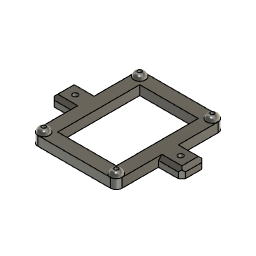
ELE#DLC_holder (Autodesk Fusion 360 design; units mm, degrees)
Autodesk Fusion 360 part; units mm, degrees
sketch "Sketch1" plane through (0, 0, 0) normal (0, 0, 1) x (1, 0, 0)
  line L0 (0, 0) -> (70, 0)
  line L1 (70, 0) -> (70, 90)
  line L2 (70, 90) -> (0, 90)
  line L3 (0, 90) -> (0, 0)
  line L4 (66.000001, 90) -> (4.000001, 90)
  line L5 (0, 90) -> (0, 86.000001)
  line L6 (0, 86.000001) -> (0, 4.000001)
  line L7 (0, 86.000001) -> (70, 86.000001)
  line L8 (66.000001, 90) -> (66.000001, 86.000001)
  line L9 (66.000001, 84.000001) -> (66.000001, 0)
  line L10 (4, 86.000001) -> (4, 0)
  line L11 (0, 4.000001) -> (4, 4.000001)
  line L12 (66.000001, 4) -> (70, 4)
  circle A0 centre (4, 86.000001) radius 1.75
  circle A1 centre (66.000001, 86.000001) radius 1.75
  circle A2 centre (66.000001, 4) radius 1.75
  circle A3 centre (4, 4.000001) radius 1.75
  dimension "d1" = 70
  dimension "d2" = 90
  dimension "d5" = 3.5
  dimension "d6" = 3.5
  dimension "d7" = 3.5
  dimension "d8" = 3.5
  constraint horizontal L0
  constraint vertical L1
  constraint horizontal L2
  constraint vertical L3
  constraint coincident L0.start L3.end
  constraint perpendicular L1 L4
  constraint perpendicular L2 L6
  constraint perpendicular L1 L7
  constraint perpendicular L7 L8
  constraint perpendicular L0 L9
  constraint coincident L0 L10.end
  constraint perpendicular L0 L10
  constraint perpendicular L10 L11
  constraint coincident L1 L12.end
  constraint perpendicular L1 L12
  measures "d1" distance of L0.start L0.end
  measures "d2" distance of L0.start L2.end
  measures "d5" diameter of A0
  measures "d6" diameter of A1
  measures "d7" diameter of A2
  measures "d8" diameter of A3
extrude "Extrude1" add sketch "Sketch1" along normal blind 8 contours L0 L3 L10 L11 A3 | L0 L1 L7 L9 L10 L12 A0 A1 A2 A3 | L3 L6 L7 L10 L11 A0 A3 | L0 L1 L9 L12 A2 | L2 L3 L4 L5 L7 L8 A0 A1 | L1 L2 L7 L8 A1 picked at (2.351293, 0.842603) picked at (25.066969, 58.2106) picked at (1.091008, 58.136049) picked at (67.648708, 0.842602) picked at (25.192233, 88.919766) picked at (69.157398, 87.648708)
sketch "Sketch2" plane through (0, 0, 0) normal (0, 0, -1) x (1, 0, 0)
  circle A0 centre (66.000001, -86.000001) radius 1.75
  circle A1 centre (4, -4.000001) radius 1.75
  circle A2 centre (4, -86.000001) radius 1.75
  circle A3 centre (66.000001, -4) radius 1.75
  line L0 (0, 0) -> (0, -90)
  line L1 (0, -90) -> (70, -90)
  line L2 (70, -90) -> (70, 0)
  line L3 (70, 0) -> (0, 0)
  line L4 (6.8, -2.383421) -> (4, -0.76684)
  line L5 (4, -0.76684) -> (1.2, -2.383421)
  line L6 (1.2, -2.383421) -> (1.2, -5.616582)
  line L7 (1.2, -5.616582) -> (4, -7.233163)
  line L8 (4, -7.233163) -> (6.8, -5.616582)
  line L9 (6.8, -5.616582) -> (6.8, -2.383421)
  line L10 (63.200001, -5.616581) -> (66.000001, -7.233162)
  line L11 (66.000001, -7.233162) -> (68.800001, -5.616581)
  line L12 (68.800001, -5.616581) -> (68.800001, -2.383419)
  line L13 (68.800001, -2.383419) -> (66.000001, -0.766839)
  line L14 (66.000001, -0.766839) -> (63.200001, -2.383419)
  line L15 (63.200001, -2.383419) -> (63.200001, -5.616581)
  line L16 (63.200001, -87.616582) -> (66.000001, -89.233163)
  line L17 (66.000001, -89.233163) -> (68.800001, -87.616582)
  line L18 (68.800001, -87.616582) -> (68.800001, -84.383421)
  line L19 (68.800001, -84.383421) -> (66.000001, -82.76684)
  line L20 (66.000001, -82.76684) -> (63.200001, -84.383421)
  line L21 (63.200001, -84.383421) -> (63.200001, -87.616582)
  line L22 (6.8, -84.383421) -> (4, -82.76684)
  line L23 (4, -82.76684) -> (1.2, -84.383421)
  line L24 (1.2, -84.383421) -> (1.2, -87.616582)
  line L25 (1.2, -87.616582) -> (4, -89.233163)
  line L26 (4, -89.233163) -> (6.8, -87.616582)
  line L27 (6.8, -87.616582) -> (6.8, -84.383421)
  point P0 (4, -4.000001)
  point P1 (66.000001, -4)
  point P2 (66.000001, -86.000001)
  point P3 (4, -86.000001)
  dimension "d11" = 2.8
  dimension "d12" = 2.8
  dimension "d13" = 2.8
  dimension "d14" = 2.8
extrude "Extrude2" cut sketch "Sketch2" against normal blind 8 contours A2 | L4 L5 L6 L7 L8 L9 | L10 L11 L12 L13 L14 L15 | L16 L17 L18 L19 L20 L21 | L22 L23 L24 L25 L26 L27 picked at (4.363702, -86.962267) picked at (5.225, -1.878239) picked at (64.775001, -1.878238) picked at (64.775001, -88.121764) picked at (2.775, -83.878239)
extrude "Extrude3" add 1 faces at (46.666667, 90, 5.333333) along direction (0, 1, 0) blind 1
extrude "Extrude4" add 1 faces at (70, 30.333333, 2.666667) along direction (1, 0, 0) blind 1
extrude "Extrude5" add 1 faces at (0, 30.333333, 2.666667) along direction (-1, 0, 0) blind 1
extrude "Extrude6" add 1 faces at (23, 0, 5.333333) along direction (0, -1, 0) blind 1
sketch "Sketch3" plane through (0, 0, 0) normal (0, 0, -1) x (1, 0, 0)
  line L0 (4, -0.76684) -> (6.8, -2.383421)
  line L1 (6.8, -2.383421) -> (6.8, -5.616582)
  line L2 (6.8, -5.616582) -> (4, -7.233163)
  line L3 (4, -7.233163) -> (1.2, -5.616582)
  line L4 (1.2, -5.616582) -> (1.2, -2.383421)
  line L5 (1.2, -2.383421) -> (4, -0.76684)
  line L6 (4, -82.76684) -> (6.8, -84.383421)
  line L7 (6.8, -84.383421) -> (6.8, -87.616582)
  line L8 (6.8, -87.616582) -> (4, -89.233163)
  line L9 (4, -89.233163) -> (1.2, -87.616582)
  line L10 (1.2, -87.616582) -> (1.2, -84.383421)
  line L11 (1.2, -84.383421) -> (4, -82.76684)
  line L12 (66.000001, -7.233162) -> (63.200001, -5.616581)
  line L13 (63.200001, -5.616581) -> (63.200001, -2.383419)
  line L14 (63.200001, -2.383419) -> (66.000001, -0.766839)
  line L15 (66.000001, -0.766839) -> (68.800001, -2.383419)
  line L16 (68.800001, -2.383419) -> (68.800001, -5.616581)
  line L17 (68.800001, -5.616581) -> (66.000001, -7.233162)
  line L18 (66.000001, -89.233163) -> (63.200001, -87.616582)
  line L19 (63.200001, -87.616582) -> (63.200001, -84.383421)
  line L20 (63.200001, -84.383421) -> (66.000001, -82.76684)
  line L21 (66.000001, -82.76684) -> (68.800001, -84.383421)
  line L22 (68.800001, -84.383421) -> (68.800001, -87.616582)
  line L23 (68.800001, -87.616582) -> (66.000001, -89.233163)
  line L24 (-1, -91) -> (71, -91)
  line L25 (71, -91) -> (71, 1)
  line L26 (71, 1) -> (-1, 1)
  line L27 (-1, 1) -> (-1, -91)
  line L28 (-1, -91) -> (71, 1)
  line L29 (35, -45) -> (35, -15)
  line L30 (35, -15) -> (60.000001, -15)
  line L31 (60.000001, -15) -> (60.000001, -75)
  line L32 (60.000001, -75) -> (10, -75)
  line L33 (10, -75) -> (10, -15)
  line L34 (10, -15) -> (35, -15)
  dimension "d25" = 60
  dimension "d26" = 60
  constraint coincident L24.start L27.end
  constraint coincident L25.end L26.start
  constraint midpoint L28 L29.start
  constraint parallel L16 L29
  constraint perpendicular L16 L30
  constraint perpendicular L30 L31
  constraint perpendicular L31 L32
  constraint perpendicular L32 L33
  constraint perpendicular L29 L34
  measures "d26" distance of L32.end L33.end
extrude "Extrude7" cut sketch "Sketch3" against normal blind 8 contours L28 L29 L32 L33 L34 | L28 L30 L31 L32 | L28 L29 L30 picked at (18.333333, -45) picked at (35.507247, -65) picked at (42.826087, -25)
sketch "Sketch4" plane through (0, 0, 8) normal (0, 0, 1) x (-1, 0, 0)
  line L0 (-10, -75) -> (-60.000001, -75)
  line L1 (-60.000001, -75) -> (-60.000001, -15)
  line L2 (-60.000001, -15) -> (-10, -15)
  line L3 (-10, -15) -> (-10, -75)
  line L4 (-6.8, -2.383421) -> (-4, -0.76684)
  line L5 (-4, -0.76684) -> (-1.2, -2.383421)
  line L6 (-1.2, -2.383421) -> (-1.2, -5.616582)
  line L7 (-1.2, -5.616582) -> (-4, -7.233163)
  line L8 (-4, -7.233163) -> (-6.8, -5.616582)
  line L9 (-6.8, -5.616582) -> (-6.8, -2.383421)
  line L10 (-6.8, -84.383421) -> (-4, -82.76684)
  line L11 (-4, -82.76684) -> (-1.2, -84.383421)
  line L12 (-1.2, -84.383421) -> (-1.2, -87.616582)
  line L13 (-1.2, -87.616582) -> (-4, -89.233163)
  line L14 (-4, -89.233163) -> (-6.8, -87.616582)
  line L15 (-6.8, -87.616582) -> (-6.8, -84.383421)
  line L16 (-63.200001, -5.616581) -> (-66.000001, -7.233162)
  line L17 (-66.000001, -7.233162) -> (-68.800001, -5.616581)
  line L18 (-68.800001, -5.616581) -> (-68.800001, -2.383419)
  line L19 (-68.800001, -2.383419) -> (-66.000001, -0.766839)
  line L20 (-66.000001, -0.766839) -> (-63.200001, -2.383419)
  line L21 (-63.200001, -2.383419) -> (-63.200001, -5.616581)
  line L22 (-63.200001, -87.616582) -> (-66.000001, -89.233163)
  line L23 (-66.000001, -89.233163) -> (-68.800001, -87.616582)
  line L24 (-68.800001, -87.616582) -> (-68.800001, -84.383421)
  line L25 (-68.800001, -84.383421) -> (-66.000001, -82.76684)
  line L26 (-66.000001, -82.76684) -> (-63.200001, -84.383421)
  line L27 (-63.200001, -84.383421) -> (-63.200001, -87.616582)
  line L28 (-71, 1) -> (-71, -91)
  line L29 (-71, -91) -> (1, -91)
  line L30 (1, -91) -> (1, 1)
  line L31 (1, 1) -> (-71, 1)
  circle A0 centre (-4, -86.000001) radius 5
  circle A1 centre (-66.000001, -86.000001) radius 4.999999
  circle A2 centre (-66.000001, -4) radius 5
  circle A3 centre (-4, -4) radius 5
  constraint tangent L30 A0
  constraint tangent L28 A1
  constraint tangent L30 A3
extrude "Extrude8" add sketch "Sketch4" along normal blind 4 contours A2 | A1 | A3 | A0 picked at (-64.233334, -7.059957) picked at (-69.533334, -86.000001) picked at (-0.466667, -4.000001) picked at (-0.466667, -86.000001)
extrude "Extrude9" cut 1 faces at (26.666667, 15, 2.666667) along direction (0, -1, 0) blind 5
extrude "Extrude10" cut 1 faces at (43.333334, 75, 2.666667) along direction (0, 1, 0) blind 5
fillet "Fillet1" radius 5 1 edges at (-1, -1, 4)
fillet "Fillet2" radius 5 1 edges at (71, -1, 4)
fillet "Fillet3" radius 5 1 edges at (71, 91, 4)
fillet "Fillet4" radius 5 1 edges at (-1, 91, 4)
sketch "Sketch5" plane through (0, 0, 12) normal (0, 0, 1) x (-1, 0, 0)
  line L0 (-4, -89.233163) -> (-6.8, -87.616582)
  line L1 (-6.8, -87.616582) -> (-6.8, -84.383421)
  line L2 (-6.8, -84.383421) -> (-4, -82.76684)
  line L3 (-4, -82.76684) -> (-1.2, -84.383421)
  line L4 (-1.2, -84.383421) -> (-1.2, -87.616582)
  line L5 (-1.2, -87.616582) -> (-4, -89.233163)
  circle A0 centre (-4, -86.000001) radius 5
  circle A1 centre (-4, -86.000001) radius 1.65
  dimension "d39" = 3.3
  constraint concentric A0 A1
  measures "d39" diameter of A1
extrude "Extrude11" add sketch "Sketch5" against normal blind 5 contours L0 L1 L2 L3 L4 L5 picked at (-5.208333, -88.092896)
extrude "Extrude12" add 1 faces at (5.208333, 88.092896, 7) along direction (0, 0, -1) blind 3
sketch "Sketch6" plane through (0, 0, 12) normal (0, 0, 1) x (-1, 0, 0)
  line L0 (-4, -7.233163) -> (-6.8, -5.616582)
  line L1 (-6.8, -5.616582) -> (-6.8, -2.383421)
  line L2 (-6.8, -2.383421) -> (-4, -0.76684)
  line L3 (-4, -0.76684) -> (-1.2, -2.383421)
  line L4 (-1.2, -2.383421) -> (-1.2, -5.616582)
  line L5 (-1.2, -5.616582) -> (-4, -7.233163)
  circle A0 centre (-4, -4) radius 5
  circle A1 centre (-4, -4) radius 1.65
  dimension "d44" = 3.3
  constraint concentric A0 A1
  measures "d44" diameter of A1
extrude "Extrude13" add sketch "Sketch6" against normal blind 8 contours L0 L1 L2 L3 L4 L5 picked at (-5.208333, -6.092896)
sketch "Sketch7" plane through (0, 0, 12) normal (0, 0, 1) x (-1, 0, 0)
  line L0 (-66.000001, -0.766839) -> (-63.200001, -2.383419)
  line L1 (-63.200001, -2.383419) -> (-63.200001, -5.616581)
  line L2 (-63.200001, -5.616581) -> (-66.000001, -7.233162)
  line L3 (-66.000001, -7.233162) -> (-68.800001, -5.616581)
  line L4 (-68.800001, -5.616581) -> (-68.800001, -2.383419)
  line L5 (-68.800001, -2.383419) -> (-66.000001, -0.766839)
  circle A0 centre (-66.000001, -4) radius 5
  circle A1 centre (-66.000001, -4) radius 1.65
  dimension "d47" = 3.3
  constraint concentric A0 A1
  measures "d47" diameter of A1
extrude "Extrude14" add sketch "Sketch7" against normal blind 8 contours L0 L1 L2 L3 L4 L5 picked at (-64.791668, -1.907105)
sketch "Sketch8" plane through (0, 0, 12) normal (0, 0, 1) x (-1, 0, 0)
  line L0 (-66.000001, -82.76684) -> (-63.200001, -84.383421)
  line L1 (-63.200001, -84.383421) -> (-63.200001, -87.616582)
  line L2 (-63.200001, -87.616582) -> (-66.000001, -89.233163)
  line L3 (-66.000001, -89.233163) -> (-68.800001, -87.616582)
  line L4 (-68.800001, -87.616582) -> (-68.800001, -84.383421)
  line L5 (-68.800001, -84.383421) -> (-66.000001, -82.76684)
  circle A0 centre (-66.000001, -86.000001) radius 4.999999
  circle A1 centre (-66.000001, -86.000001) radius 1.65
  dimension "d50" = 3.3
  constraint concentric A0 A1
  measures "d50" diameter of A1
extrude "Extrude15" add sketch "Sketch8" against normal blind 8 contours L0 L1 L2 L3 L4 L5 picked at (-63.583334, -86.000001)
fillet "Fillet5" radius 4 1 edges at (70.661638, 5.808077, 12)
fillet "Fillet6" radius 4 3 edges at (8.661637, 5.808077, 12) (8.661637, 87.808078, 12) (70.661637, 87.808078, 12)
sketch "Sketch9" plane through (-1, 0, 0) normal (-1, 0, 0) x (0, -1, 0)
  line L0 (-86.000001, 8) -> (-86, 0)
  line L1 (-86, 0) -> (-4, 0)
  line L2 (-4, 0) -> (-4, 8)
  line L3 (-4, 8) -> (-86.000001, 8)
  line L4 (-86.000001, 8) -> (-4, 0)
  line L5 (-45.000001, 4) -> (-45.000001, 8)
  line L6 (-45.000001, 8) -> (-55.000001, 8)
  line L7 (-45.000001, 8) -> (-35.000001, 8)
  line L8 (-35.000001, 8) -> (-55.000001, 8)
  line L9 (-55.000001, 8) -> (-55.000001, 0)
  line L10 (-55.000001, 0) -> (-35.000001, 0)
  line L11 (-35.000001, 0) -> (-35.000001, 8)
  constraint coincident L1.end L2.start
  constraint parallel L3 L6
  constraint parallel L3 L7
  constraint horizontal L8
  constraint vertical L9
  constraint horizontal L10
  constraint vertical L11
extrude "Extrude16" add sketch "Sketch9" along normal blind 10 contours L3 L4 L5 L6 L8 L9 | L1 L4 L9 L10 L11 | L3 L4 L5 L7 L8 L11 picked at (-48.333334, 5.658537) picked at (-51.666667, 2.99187) picked at (-38.333334, 5.00813)
extrude "Extrude17" add 1 faces at (-11, 48.333334, 5.333333) along direction (-1, 0, 0) blind 10
sketch "Sketch10" plane through (0, 0, 8) normal (0, 0, 1) x (-1, 0, 0)
  arc A0 (-66.000001, -91) -> (-71, -86.000001) centre (-66.000001, -86.000001) ccw
  line L0 (-66.000001, -91) -> (-4, -91)
  arc A1 (1, -86.000001) -> (-4, -91.000001) centre (-4, -86.000001) ccw
  line L1 (1, -86.000001) -> (1, -55.000001)
  line L2 (1, -55.000001) -> (21, -55.000001)
  line L3 (21, -55.000001) -> (21, -35.000001)
  line L4 (21, -35.000001) -> (1, -35.000001)
  line L5 (1, -35.000001) -> (1, -4)
  arc A2 (-4, 1) -> (1, -4) centre (-4, -4) ccw
  line L6 (-4, 1) -> (-66.000001, 1)
  arc A3 (-71.000001, -4) -> (-66.000001, 1) centre (-66.000001, -4) ccw
  line L7 (-71.000001, -4) -> (-71, -86.000001)
  line L8 (-10, -10) -> (-10, -80)
  line L9 (-10, -80) -> (-60.000001, -80)
  line L10 (-60.000001, -80) -> (-60.000001, -10)
  line L11 (-60.000001, -10) -> (-10, -10)
  circle A4 centre (10, -45.000001) radius 2.2
  line L12 (-10, -45) -> (-60.000001, -45)
  line L13 (-60.000001, -45) -> (-80.000001, -45)
  circle A5 centre (-80.000001, -45) radius 2.2
  line L14 (-71, -55.000001) -> (-91, -55.000001)
  line L15 (-91, -55.000001) -> (-91, -35.000001)
  line L16 (-91, -35.000001) -> (-71, -35.000001)
  line L17 (-71, -35.000001) -> (-71, -55.000001)
  dimension "d59" = 4.4
  dimension "d60" = 20
  dimension "d61" = 4.4
  dimension "d62" = 20
  dimension "d63" = 20
  constraint midpoint L8 L12.start
  constraint perpendicular L7 L13
  constraint horizontal L14
  constraint vertical L15
  constraint horizontal L16
  constraint vertical L17
  measures "d59" diameter of A4
  measures "d61" diameter of A5
extrude "Extrude18" add sketch "Sketch10" against normal blind 8 contours L7 L14 L15 L16 L17 picked at (-88.066667, -45.000001)
extrude "Extrude19" cut sketch "Sketch10" against normal blind 8 contours A4 picked at (10.6851, -45.425038)
chamfer "Chamfer1" distance 3 angle 45 6 edges at (81, 55.000001, 8) (91, 45.000001, 8) (81, 35.000001, 8) (-11, 55.000001, 8) (-21, 45.000001, 8) (-11, 35.000001, 8)
chamfer "Chamfer2" distance 3 angle 45 2 edges at (91, 55.000001, 2.5) (-21, 55.000001, 2.5)
chamfer "Chamfer3" distance 3 angle 45 2 edges at (-21, 35.000001, 2.5) (91, 35.000001, 2.5)
equation "d11 = ( 5.6 / 2 ) * 1 mm"
equation "d12 = ( 5.6 / 2 ) * 1 mm"
